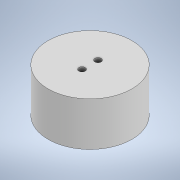
# Autodesk Inventor part: motor_subsitude
Saved by Autodesk Inventor 2020.1 (Build 241239000, 239)
## iProperties
Created: 2021-08-15
Part Number: motor_subsitude
Material: Generic
Document SubType Name: Modeling
Designer: Mic
Density: 1 g/cm^3
Appearance: Default
Author: Mic
Autodesk Inventor part; units mm, degrees
ref_plane "YZ Plane" through (0, 0, 0) normal (1, 0, 0) x (0, 1, 0)
ref_plane "XZ Plane" through (0, 0, 0) normal (0, 1, 0) x (-1, 0, 0)
ref_plane "XY Plane" through (0, 0, 0) normal (0, 0, 1) x (1, 0, 0)
sketch "Sketch1" plane through (0, 0, 0) normal (0, 1, 0) x (-1, 0, 0)
  circle A0 centre (0, 0) radius 6 construction
  circle A1 centre (6, 0) radius 1
  circle A2 centre (0, 6) radius 1
  circle A3 centre (-6, 0) radius 1
  circle A4 centre (0, -6) radius 1
  circle A5 centre (0, 0) radius 13.1
  dimension "d0" = 12
  dimension "d1" = 2
  dimension "d2" = 2
  dimension "d3" = 2
  dimension "d4" = 2
  dimension "d10" = 26.2
  constraints: 6 centre point, 4 point on circle, 2 coincident
  measures "d0" diameter of A0
  measures "d1" diameter of A1
  measures "d2" diameter of A2
  measures "d3" diameter of A3
  measures "d4" diameter of A4
  measures "d10" diameter of A5
extrude "Extrusion1" add sketch "Sketch1" along normal blind 6
sketch "Sketch2" plane through (0, 6, 0) normal (0, 1, 0) x (1, 0, 0)
  circle A0 centre (0, 0) radius 13.1 projected
  circle A1 centre (0, 0) radius 2.5 construction
  circle A2 centre (0, -2.5) radius 1
  circle A3 centre (0, 2.5) radius 1
  dimension "d7" = 5
  dimension "d8" = 2
  dimension "d9" = 2
  constraints: 3 centre point, 2 point on circle, 1 coincident
  measures "d7" diameter of A1
  measures "d8" diameter of A2
  measures "d9" diameter of A3
extrude "Extrusion2" add sketch "Sketch2" along normal blind 7.7
body "Solid1"
